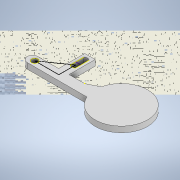
# Autodesk Inventor part: PINZA_D
Saved by Autodesk Inventor 2022 (Build 260153000, 153)
## iProperties
Created: 2022-11-02
Part Number: PINZA_D
Material: Genérico
Document SubType Name: Modeling
Designer: Usuario
Density: 1 g/cm^3
Appearance: Valor por defecto
Author: Usuario
Autodesk Inventor part; units mm, degrees
note: some values were not read from the file. Chosen so that the rebuilt part matches the saved one: second side of "Extrusión2".
ref_plane "YZ Plane" through (0, 0, 0) normal (1, 0, 0) x (0, 1, 0)
ref_plane "XZ Plane" through (0, 0, 0) normal (0, 1, 0) x (-1, 0, 0)
ref_plane "XY Plane" through (0, 0, 0) normal (0, 0, 1) x (1, 0, 0)
sketch "Boceto1" plane through (0, 0, 0) normal (0, 1, 0) x (-1, 0, 0)
  line L0 (50, 10) -> (-50, 10)
  line L1 (-50, 10) -> (-50, -10)
  line L2 (-50, -10) -> (50, -10)
  line L3 (50, -10) -> (50, 10)
  line L4 (50, 10) -> (-50, -10) construction
  line L5 (-50, 10) -> (50, -10) construction
  line L6 (-50, -10) -> (-20, -10)
  line L7 (-20, -10) -> (0, 0)
  line L8 (0, 0) -> (50, 0)
  line L9 (0, 0) -> (0, 10)
  dimension "d0" = 100
  dimension "d1" = 20
  dimension "d2" = 30
  constraints: 20 end point, 4 midpoint, 2 parallel, 1 horizontal, 1 perpendicular, 1 point on line
  measures "d0" distance of L2.end L1.end
  measures "d1" distance of L1.end L0.end
  measures "d2" distance of L1.end L6.end
extrude "Extrusión1" add sketch "Boceto1" along normal blind 5.5 contours L3 L8 L9 L0
extrude "Extrusión2" add sketch "Boceto1" along normal blind 5.5 contours L9 L7 L2 L1 L0
sketch "Boceto2" plane through (0, 5.5, 0) normal (0, 1, 0) x (1, 0, 0)
  line L0 (-50, 0) -> (-50, -10) projected
  line L1 (-50, -10) -> (-45, -10)
  line L2 (-50, -10) -> (50, -10) projected
  line L3 (-45, -10) -> (-45, 0)
  line L4 (0, 0) -> (-50, 0) projected
  arc A0 (-45, 0) -> (-45, -10) centre (-45, -5) ccw
  line L5 (-50, -5) -> (-25, -5)
  line L6 (-25, -5) -> (-25, 25)
  line L7 (-25, 25) -> (-15, 25)
  line L8 (-15, 25) -> (-15, -5)
  line L9 (-15, -5) -> (-25, -5)
  line L10 (-20, 25) -> (-20, 5)
  line L11 (-22.5, 7.5) -> (-17.5, 7.5)
  line L12 (-17.5, 7.5) -> (-17.5, 22.5)
  line L13 (-17.5, 22.5) -> (-22.5, 22.5)
  line L14 (-22.5, 22.5) -> (-22.5, 7.5)
  line L15 (-22.5, 7.5) -> (-17.5, 22.5) construction
  line L16 (-17.5, 7.5) -> (-22.5, 22.5) construction
  line L17 (-22.5, 22.5) -> (-22.5, 21.5)
  line L18 (-22.5, 21.5) -> (-17.5, 21.5)
  line L19 (-22.5, 15) -> (-17.5, 15)
  arc A1 (-17.5, 21.5) -> (-22.5, 21.5) centre (-20, 18.875) ccw
  arc A2 (-22.5, 8.5) -> (-17.5, 8.5) centre (-20, 11.125) ccw
  line L20 (-25, -5) -> (-20, -5)
  line L21 (-20, -5) -> (-20, -10)
  line L22 (-20, -10) -> (-25, -10)
  line L23 (-25, -10) -> (-25, -5)
  point P0 (0, -10)
  point P1 (-20, 15)
  point P2 (-50, -5)
  point P3 (-25, 0)
  point P4 (-15, 0)
  point P5 (-20, 22.5)
  point P6 (-20, 7.5)
  point P7 (-22.5, 8.5)
  point P8 (-17.5, 8.5)
  point P9 (-20, -5)
  dimension "d7" = 5
  dimension "d8" = 25
  dimension "d9" = 30
  dimension "d10" = 10
  dimension "d11" = 20
  dimension "d12" = 5
  dimension "d13" = 15
  dimension "d14" = 1
  constraints: 42 end point, 8 perpendicular, 7 point on circle, 6 midpoint, 6 point on line, 4 parallel, 3 centre point, 3 horizontal, 3 symmetric about line, 2 tangent, 1 vertical, 1 other
  measures "d7" distance of L0.end L1.end
  measures "d8" distance of L5.start L5.end
  measures "d9" distance of L5.end L6.end
  measures "d10" distance of L6.end L7.end
  measures "d11" distance of L10.start L10.end
  measures "d12" distance of L13.end L12.end
  measures "d13" distance of L12.end L11.end
  measures "d14" distance of L13.end L17.end
extrude "Extrusión3" cut sketch "Boceto2" against normal blind 5.5 contours L4 A0 L0 | A0 L1 L0
extrude "Extrusión4" add sketch "Boceto2" against normal blind 5.5 contours L6 L7 L8 L4 | L4 L8 L9 L6
extrude "Extrusión5" add sketch "Boceto2" against normal blind 5.5 contours A1 L14 L13 | L13 L12 A1 | A2 L12 L11 | L11 L14 A2
sketch "Boceto3" plane through (0, 5.5, 0) normal (0, 1, 0) x (1, 0, 0)
  arc A0 (-45, 0) -> (-45, -10) centre (-45, -5) ccw projected
  line L0 (-45, -5) -> (-43, -5)
  circle A1 centre (-43, -5) radius 3
  point P0 (0, 0)
  dimension "d21" = 2
  dimension "d22" = 6
  constraints: 2 end point, 1 centre point, 1 coincident, 1 horizontal
  measures "d21" distance of L0.start L0.end
  measures "d22" diameter of A1
extrude "Extrusión6" cut sketch "Boceto3" against normal blind 5.5
sketch "Boceto4" plane through (0, 5.5, 0) normal (0, 1, 0) x (1, 0, 0)
  line L0 (0, 0) -> (50, 0)
  line L1 (50, -10) -> (50, 10) projected
  line L2 (50, 10) -> (20, 10) projected
  line L3 (20, 10) -> (20, 0)
  line L4 (50, 0) -> (20, 0)
  circle A0 centre (35, 0) radius 25
  dimension "d27" = 50
  constraints: 6 end point, 2 midpoint, 2 perpendicular, 1 centre point, 1 point on line
  measures "d27" diameter of A0
extrude "Extrusión7" add sketch "Boceto4" against normal blind 5.5
sketch "Boceto5" plane through (0, 5.5, 0) normal (0, 1, 0) x (1, 0, 0)
  line L0 (-22.5, 8.5) -> (-22.5, 21.5) projected
  arc A0 (-22.5, 8.5) -> (-17.5, 8.5) centre (-20, 11.125) ccw projected
  line L1 (-17.5, 21.5) -> (-17.5, 8.5) projected
  circle A1 centre (-43, -5) radius 3 projected
  line L2 (-43, -5) -> (-20, -5)
  line L3 (-20, -5) -> (-20, 11.125)
  line L4 (-20, 11.125) -> (-43, -5)
  line L5 (-22.5, 13.75) -> (-17.5, 13.75)
  point P0 (0, 0)
  constraints: 8 end point, 2 perpendicular, 2 point on line, 1 horizontal
